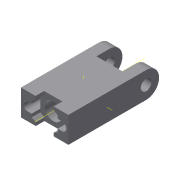
# Autodesk Inventor part: empty
Saved by Autodesk Inventor 2014 (Build 180170000, 170)
## iProperties
Created: 2015-04-13
Part Number: empty
Material: Generic
Document SubType Name: Modeling
Designer: Martin
Density: 1 g/cm^3
Appearance: Default
Mass: 0.578402 g
Surface Area: 7.54528 cm^2
Volume: 0.578402 cm^3
Author: Martin
Autodesk Inventor part; units mm, degrees
ref_plane "plane_support" through (-5.5, -8, -3) normal (0, -1, 0) x (1, 0, 0)
ref_plane "plane_support_frontb" through (-2.5, 0, 0) normal (1, 0, 0) x (0, 0, -1)
ref_plane "plane_support_frontt" through (2.5, 0, 0) normal (-1, 0, 0) x (0, 0, 1)
sketch "Sketch14" plane through (0, 0, 0) normal (1, 0, 0) x (0, 1, 0)
  line L0 (-13.2, 0) -> (16.2, 0) projected
  line L1 (0, -4.2) -> (0, 4.2) projected
  line L2 (9, -3) -> (-9, -3)
  line L3 (-9, -3) -> (-9, 3)
  line L4 (-9, 3) -> (9, 3)
  line L5 (9, 3) -> (9, -3) construction
  line L6 (9, -3) -> (-9, 3) construction
  line L7 (-9, -3) -> (9, 3) construction
  line L8 (5.5, 3) -> (5.5, -3) construction
  line L9 (-6.5, 3) -> (-6.5, -3) construction
  arc A0 (9, -3) -> (9, 3) centre (9, 0) ccw
  circle A1 centre (9, 0) radius 1.25
  circle A2 centre (9, 0) radius 3 construction
  line L10 (6, 3) -> (6, -3) construction
  point P0 (0, 0)
  point P1 (0, 0)
  dimension "d72" = 6
  dimension "d73" = 12
  dimension "d74" = 2.5
  dimension "d75" = 2.5
  dimension "d76" = 0.5
  constraints: 18 end point, 6 point on line, 4 perpendicular, 3 centre point, 3 midpoint, 3 tangent, 2 coincident, 2 parallel, 2 point on circle, 1 concentric, 1 horizontal
  measures "d72" distance between parallel lines of L2 L4
  measures "d73" distance between parallel lines of L8 L9
  measures "d74" distance between parallel lines of L3 L9
  measures "d75" diameter of A1
  measures "d76" distance between parallel lines of L8 L10
extrude "ext_main" add sketch "Sketch14" along normal mid plane 11 contours L3 L4 L1 L0 | L0 L1 L2 L3 | L1 L4 A0 L0 A1 | L0 A1 A0 L2 L1
sketch "Sketch15" plane through (0, 0, 0) normal (1, 0, 0) x (0, 1, 0)
  circle A0 centre (9, 0) radius 1.25 projected
  arc A1 (9, -3) -> (9, 3) centre (9, 0) ccw projected
  circle A2 centre (9, 0) radius 3
  line L0 (6, 3) -> (6, -3)
  line L1 (9, 3) -> (-9, 3) projected
  line L2 (-9, -3) -> (9, -3) projected
  line L3 (-13.2, 0) -> (16.2, 0) projected
  point P0 (0, 0)
  constraints: 2 end point, 2 point on line, 1 centre point, 1 coincident, 1 concentric, 1 perpendicular, 1 tangent
extrude "ext_cut_front" cut sketch "Sketch15" along normal mid plane 6 contours L3 A1 A2 A0 | A0 L3 A2 A1 | L0 L1 A2 | A2 L2 L0
sketch "sk_channel_nut" plane through (-5.5, -9, -3) normal (0, -1, 0) x (1, 0, 0)
  line L0 (-2.2, 3) -> (13.2, 3) projected
  line L1 (5.5, -1.8497) -> (5.5, 7.8497) projected
  circle A0 centre (5.5, 3) radius 2
  line L2 (5.5, 6.4641) -> (2.5, 4.7321)
  line L3 (2.5, 4.7321) -> (2.5, 1.2679)
  line L4 (2.5, 1.2679) -> (5.5, -0.4641)
  line L5 (5.5, -0.4641) -> (8.5, 1.2679)
  line L6 (8.5, 1.2679) -> (8.5, 4.7321)
  line L7 (8.5, 4.7321) -> (5.5, 6.4641)
  circle A1 centre (1.5, 3) radius 1
  circle A2 centre (9.5, 3) radius 1
  line L8 (1.5, 4) -> (2.5, 4)
  line L9 (1.5, 2) -> (2.5, 2)
  line L10 (9.5, 4) -> (8.5, 4)
  line L11 (9.5, 2) -> (8.5, 2)
  line L12 (11, 0) -> (0, 0) projected
  line L13 (11, 6) -> (0, 6) projected
  line L14 (0, 0) -> (0, 6) projected
  line L15 (3.4, 6) -> (3.4, 5.2517)
  line L16 (3.4456, 0.722) -> (3.4456, 0)
  line L17 (7.5544, 0.722) -> (7.5544, 0)
  line L18 (7.6, 6) -> (7.6, 5.2517)
  point P0 (5.5, 3)
  point P1 (2.5, 3)
  dimension "d85" = 4
  dimension "d86" = 120
  dimension "d87" = 6
  dimension "d88" = 2
  dimension "d95" = 4.2
  constraints: 28 end point, 17 point on line, 7 parallel, 5 equal length, 5 point on circle, 5 tangent, 3 centre point, 3 perpendicular, 1 coincident, 1 equal radius, 1 midpoint, 2 other
  measures "d85" diameter of A0
  measures "d86" angle of L7 L2
  measures "d87" distance between parallel lines of L3 L6
  measures "d88" diameter of A1
  measures "d95" distance between parallel lines of L18 L15
extrude "ext_cut_channel" cut sketch "sk_channel_nut" against normal up to surface (15 mm away) contours A0 L1 L0 | L0 L1 A0 | L1 A0 L0 | L0 A0 L1
extrude "ext_cut_bottomscrews" cut sketch "sk_channel_nut" against normal blind 8 contours A1 L0 | L0 A1 | A1 L8 L3 | L3 L9 A1 | A2 L0 | A2 L11 L6 | L6 L10 A2 | L0 A2
extrude "ext_cut_bottom_nut" cut sketch "sk_channel_nut" against normal blind 2 contours L3 L2 L13 L1 A0 L0 | L0 A0 L1 L12 L4 L3 | L16 L4 L12 | L13 L2 L15 | A0 L1 L0 | L0 L1 A0 | L12 L1 L4 | L2 L1 L13 | L1 A0 L0 | L0 A0 L1 | L1 L13 L7 L6 L0 A0 | A0 L0 L6 L5 L12 L1 | L1 L12 L5 | L7 L13 L1 | L5 L17 L12 | L13 L18 L7
sketch "Sketch19" plane through (-5.5, -8, -3) normal (0, -1, 0) x (1, 0, 0)
  line L0 (3.4, 6) -> (7.6, 6) projected
  line L1 (3.4, 5.2517) -> (3.4, 6) projected
  line L2 (2.5, 4.7321) -> (3.4, 5.2517) projected
  line L3 (2.5, 4) -> (2.5, 4.7321) projected
  line L4 (2.5, 2) -> (2.5, 4) projected
  line L5 (2.5, 1.2679) -> (2.5, 2) projected
  line L6 (3.4456, 0.722) -> (2.5, 1.2679) projected
  line L7 (3.4456, 0) -> (3.4456, 0.722) projected
  line L8 (7.5544, 0) -> (3.4456, 0) projected
  line L9 (7.5544, 0.722) -> (7.5544, 0) projected
  line L10 (8.5, 1.2679) -> (7.5544, 0.722) projected
  line L11 (8.5, 2) -> (8.5, 1.2679) projected
  line L12 (8.5, 4) -> (8.5, 2) projected
  line L13 (8.5, 4.7321) -> (8.5, 4) projected
  line L14 (7.6, 5.2517) -> (8.5, 4.7321) projected
  line L15 (7.6, 6) -> (7.6, 5.2517) projected
  circle A0 centre (5.5, 3) radius 2 projected
  line L16 (3.9, 5.5) -> (7.1, 5.5) construction
  line L17 (7.1, 5.5) -> (7.1, 4.963)
  line L18 (7.1, 4.963) -> (8, 4.4434)
  line L19 (8, 4.4434) -> (8, 4)
  line L20 (8, 4) -> (8, 2)
  line L21 (8, 2) -> (8, 1.5566)
  line L22 (8, 1.5566) -> (7.0544, 1.0107)
  line L23 (7.0544, 1.0107) -> (7.0544, 0.5)
  line L24 (7.0544, 0.5) -> (3.9456, 0.5) construction
  line L25 (3.9456, 0.5) -> (3.9456, 1.0107)
  line L26 (3.9456, 1.0107) -> (3, 1.5566)
  line L27 (3, 1.5566) -> (3, 2)
  line L28 (3, 2) -> (3, 4)
  line L29 (3, 4) -> (3, 4.4434)
  line L30 (3, 4.4434) -> (3.9, 4.963)
  line L31 (3.9, 4.963) -> (3.9, 5.5)
  line L32 (3.9, 5.5) -> (7.1, 5.5)
  line L33 (7.1, 5.5) -> (7.1, 6)
  line L34 (7.1, 6) -> (3.9, 6)
  line L35 (3.9, 6) -> (3.9, 5.5)
  line L36 (3.9456, 0.5) -> (7.0544, 0.5)
  line L37 (7.0544, 0.5) -> (7.0544, 0)
  line L38 (7.0544, 0) -> (3.9456, 0)
  line L39 (3.9456, 0) -> (3.9456, 0.5)
  point P0 (5.5, 3)
  dimension "d97" = 0.4
  constraints: 48 end point, 6 equal length, 2 collinear, 2 perpendicular, 15 other
sketch "Sketch20" plane through (-2.5, 0, 0) normal (1, 0, 0) x (0, 0, -1)
  circle A0 centre (0, 9) radius 1.25 projected
  arc A1 (3, 9) -> (-3, 9) centre (0, 9) ccw projected
  line L0 (-3, 6) -> (-3, 9) projected
  line L1 (3, 6) -> (-3, 6) projected
  line L2 (3, 9) -> (3, 6) projected
  line L3 (-3, 7) -> (3, 7)
  point P0 (0, 0)
  dimension "d102" = 1
  constraints: 2 end point, 2 point on line, 1 perpendicular
  measures "d102" distance between parallel lines of L1 L3
equation "\"d73\" = linact_rod_effective_length"
equation "\"d74\" = nut_m3_thickness_max"
equation "\"d75\" = screw_m2_bore_loose"
equation "\"d87\" = nut_m3_width_acrossflats"
equation "\"d88\" = screw_m2_bore_selfthreading"
equation "\"d95\" = 0.7 * nut_m3_width_acrossflats"
equation "\"d89\" = linact_rod_effective_length + nut_m3_thickness_max"
equation "\"d93\" = 0.8 * nut_m3_thickness_max"
equation "\"d97\" = print_support_z_clearance"
equation "\"d102\" = print_support_xy_clearance"
equation "\"d96\" = print_support_xy_clearance"
equation "\"d100\" = print_support_z_clearance"
equation "\"d101\" = print_support_z_clearance"
equation "\"linact_rod_effective_length\" = 12"
equation "\"nut_m3_thickness_max\" = 2.5"
equation "\"screw_m2_bore_loose\" = 2.5"
equation "\"nut_m3_width_acrossflats\" = 6"
equation "\"screw_m2_bore_selfthreading\" = 2"
equation "\"print_support_z_clearance\" = 0.4"
equation "\"print_support_xy_clearance\" = 1"
body "Solid3"
